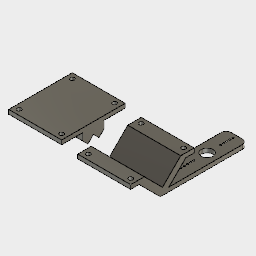
pen-arm (Autodesk Fusion 360 design; units mm, degrees)
Autodesk Fusion 360 part; units mm, degrees
sketch "Sketch1" plane through (0, 0, 0) normal (0, 0, 1) x (1, 0, 0)
  line L0 (-10, -50) -> (10, -50)
  line L1 (10, -50) -> (10, 45)
  line L2 (5, 50) -> (-5, 50)
  line L3 (-10, 45) -> (-10, -50)
  line L4 (-10, -50) -> (10, 50) construction
  line L5 (10, -50) -> (-10, 50) construction
  circle A0 centre (0.0086, 22) radius 5.5
  circle A1 centre (0.0086, 34.5) radius 0.75
  circle A2 centre (0.0086, 37.5) radius 0.75
  circle A3 centre (0.0086, 40.5) radius 0.75
  circle A4 centre (0.0086, 43.5) radius 0.75
  circle A5 centre (0.0086, 46.5) radius 0.75
  arc A6 (10, 45) -> (5, 50) centre (5, 45) ccw
  arc A7 (-5, 50) -> (-10, 45) centre (-5, 45) ccw
  circle A8 centre (0.0086, 9.5) radius 0.75
  circle A9 centre (0.0086, 6.5) radius 0.75
  circle A10 centre (0.0086, 3.5) radius 0.75
  circle A11 centre (0.0086, 0.5) radius 0.75
  circle A12 centre (0.0086, -2.5) radius 0.75
  dimension "d1" = 20
  dimension "d2" = 100
  dimension "d3" = 11
  dimension "d4" = 28
  dimension "d5" = 1.5
  dimension "d6" = 12.5
  dimension "d7" = 1.5
  dimension "d8" = 3
  dimension "d9" = 1.5
  dimension "d10" = 3
  dimension "d11" = 1.5
  dimension "d12" = 3
  dimension "d13" = 1.5
  dimension "d14" = 3
  dimension "d15" = 5
  dimension "d16" = 5
  dimension "d17" = 1.5
  dimension "d18" = 12.5
  dimension "d19" = 1.5
  dimension "d20" = 1.5
  dimension "d21" = 1.5
  dimension "d22" = 1.5
  dimension "d23" = 3
  dimension "d24" = 3
  dimension "d25" = 3
  dimension "d26" = 3
  measures "d1" distance of L4.end L5.end
  measures "d2" distance of L0.end L4.end
  measures "d3" diameter of A0
  measures "d4" distance of L2 A0.centre
  measures "d5" diameter of A1
  measures "d6" distance of A0.centre A1.centre
  measures "d7" diameter of A2
  measures "d8" distance of A1.centre A2.centre
  measures "d9" diameter of A3
  measures "d10" distance of A2.centre A3.centre
  measures "d11" diameter of A4
  measures "d12" distance of A3.centre A4.centre
  measures "d13" diameter of A5
  measures "d14" distance of A4.centre A5.centre
  measures "d15" radius of A6
  measures "d16" radius of A7
  measures "d17" diameter of A8
  measures "d18" distance of A0.centre A8.centre
  measures "d19" diameter of A9
  measures "d20" diameter of A10
  measures "d21" diameter of A11
  measures "d22" diameter of A12
  measures "d23" distance of A8.centre A9.centre
  measures "d24" distance of A9.centre A10.centre
  measures "d25" distance of A10.centre A11.centre
  measures "d26" distance of A11.centre A12.centre
extrude "Extrude1" add sketch "Sketch1" along normal blind 4 makes body 1
sketch "Sketch2" plane through (-10, 0, 0) normal (-1, 0, 0) x (0, -1, 0)
  line L0 (-45, 0) -> (50, 0)
  line L1 (50, 0) -> (50, 4)
  line L2 (50, 4) -> (-45, 4)
  line L3 (-45, 4) -> (-45, 0)
  line L4 (50, 4) -> (10, 4)
  line L5 (10, 4) -> (10, 0)
  line L6 (10, 0) -> (50, 0)
  line L7 (50, 0) -> (50, 4)
  dimension "d31" = 40
  measures "d31" distance of L1.end L4.end
extrude "Extrude2" add sketch "Sketch2" along normal blind 30 contours L0 L1 L2 L4 L5 L6 L7 bodies 1
sketch "Sketch3" plane through (0, 0, 4) normal (0, 0, 1) x (-1, 0, 0)
  circle A0 centre (-0.0086, -0.5) radius 0.75
  circle A1 centre (-0.0086, -34.5) radius 0.75
  circle A2 centre (-0.0086, -37.5) radius 0.75
  circle A3 centre (-0.0086, -40.5) radius 0.75
  circle A4 centre (-0.0086, -6.5) radius 0.75
  circle A5 centre (-0.0086, -46.5) radius 0.75
  circle A6 centre (-0.0086, -43.5) radius 0.75
  circle A7 centre (-0.0086, -9.5) radius 0.75
  circle A8 centre (-0.0086, -22) radius 5.5
  circle A9 centre (-0.0086, 2.5) radius 0.75
  circle A10 centre (-0.0086, -3.5) radius 0.75
  arc A11 (5, -50) -> (10, -45) centre (5, -45) ccw
  line L0 (10, -45) -> (10, 10)
  line L1 (10, 10) -> (40, 10)
  line L2 (40, 10) -> (40, 50)
  line L3 (40, 50) -> (-10, 50)
  line L4 (-10, 50) -> (-10, -45)
  arc A12 (-10, -45) -> (-5, -50) centre (-5, -45) ccw
  line L5 (-5, -50) -> (5, -50)
  line L6 (-10, 50) -> (40, 50)
  line L7 (40, 50) -> (40, 10)
  line L8 (40, 10) -> (-10, 10)
  line L9 (-10, 10) -> (-10, 50)
extrude "Extrude3" add sketch "Sketch3" along normal blind 20 contours L1 L2 L3 L4 L6 L7 L8 L9 bodies 1
sketch "Sketch4" plane through (0, 0, 24) normal (0, 0, 1) x (-1, 0, 0)
  line L0 (-10, 10) -> (40, 10)
  line L1 (40, 10) -> (40, 50)
  line L2 (40, 50) -> (-10, 50)
  line L3 (-10, 50) -> (-10, 10)
  line L4 (40, 30) -> (-10, 30)
split "Split1" by curves path "Sketch4" along L4 bodies 1 makes body 2 at (-6.6667, -50, 16)
draft "Draft1" angle -45 neutral plane through (-40, -50, 4) pull (0, -1, 0) 1 faces at (-6.6667, -43.3333, 24) on bodies 2
draft "Draft2" angle -45 neutral plane through (-10, -10, 4) pull (0, 1, 0) 1 faces at (-6.6667, -23.3333, 24) on bodies 1
combine "Combine1" operation add target body 2 tool bodies 1
sketch "Sketch5" plane through (0, -10, 0) normal (0, 1, 0) x (-1, 0, 0)
  line L0 (10, 4) -> (10, 0)
  line L1 (10, 0) -> (40, 0)
  line L2 (40, 0) -> (40, 24)
  line L3 (40, 24) -> (-10, 24)
  line L4 (-10, 24) -> (-10, 4)
  line L5 (-10, 4) -> (10, 4)
  line L6 (-10, 24) -> (40, 24)
  line L7 (40, 24) -> (40, 20)
  line L8 (40, 20) -> (-10, 20)
  line L9 (-10, 20) -> (-10, 24)
  dimension "d40" = 4
  measures "d40" distance of L3.end L8.end
extrude "Extrude4" add sketch "Sketch5" along normal blind 10 contours L2 L3 L4 L6 L7 L8 L9 bodies 2
sketch "Sketch6" plane through (0, -50, 0) normal (0, -1, 0) x (1, 0, 0)
  line L0 (-40, 0) -> (10, 0)
  line L1 (10, 0) -> (10, 24)
  line L2 (10, 24) -> (-40, 24)
  line L3 (-40, 24) -> (-40, 0)
  line L4 (-40, 24) -> (10, 24)
  line L5 (10, 24) -> (10, 20)
  line L6 (10, 20) -> (-40, 20)
  line L7 (-40, 20) -> (-40, 24)
  dimension "d43" = 4
  measures "d43" distance of L2.end L6.end
extrude "Extrude5" add sketch "Sketch6" along normal blind 10 contours L1 L2 L3 L4 L5 L6 L7 bodies 2
chamfer "Chamfer1" distance 2 angle 45 1 edges at (-15, -10, 20) on bodies 2
chamfer "Chamfer2" distance 2 angle 45 1 edges at (-15, -50, 20) on bodies 2
sketch "Sketch7" plane through (0, 0, 0) normal (0, 0, 1) x (1, 0, 0)
  line L0 (-49.9475, -0.0799) -> (-99.9475, -0.0799)
  line L1 (-99.9475, -0.0799) -> (-99.9475, -60.0799)
  line L2 (-99.9475, -60.0799) -> (-49.9475, -60.0799)
  line L3 (-49.9475, -60.0799) -> (-49.9475, -0.0799)
  dimension "d48" = 50
  dimension "d49" = 60
  measures "d48" distance of L0.start L0.end
  measures "d49" distance of L0.start L2.end
extrude "Extrude6" add sketch "Sketch7" along normal blind 4 separate body makes body 3
sketch "Sketch8" plane through (0, 0, 4) normal (0, 0, 1) x (-1, 0, 0)
  line L0 (49.9475, 60.0799) -> (49.9475, 0.0799)
  line L1 (49.9475, 0.0799) -> (99.9475, 0.0799)
  line L2 (99.9475, 0.0799) -> (99.9475, 60.0799)
  line L3 (99.9475, 60.0799) -> (49.9475, 60.0799)
  line L4 (99.9475, 30.0799) -> (49.9475, 30.0799)
  line L5 (99.9475, 40.0799) -> (49.9475, 40.0799)
  line L6 (99.9475, 20.0799) -> (49.9475, 20.0799)
  dimension "d52" = 10
  dimension "d53" = 10
  measures "d52" distance of L4 L5
  measures "d53" distance of L4 L6
extrude "Extrude7" add sketch "Sketch8" along normal blind 10 contours L0 L2 L4 L5 bodies 3
chamfer "Chamfer3" distance 7 angle 45 1 edges at (-74.9475, -30.0799, 14) on bodies 3
extrude "Extrude8" add sketch "Sketch8" along normal blind 10 contours L0 L2 L4 L6 bodies 3
chamfer "Chamfer4" distance 7 angle 45 1 edges at (-74.9475, -30.0799, 14) on bodies 3
sketch "Sketch9" plane through (0, 0, 24) normal (0, 0, 1) x (-1, 0, 0)
  line L0 (40, 10) -> (-10, 10)
  line L1 (-10, 10) -> (-10, 0)
  line L2 (-10, 0) -> (40, 0)
  line L3 (40, 0) -> (40, 10)
  circle A0 centre (-5, 5) radius 2
  circle A1 centre (35, 5) radius 2
  circle A2 centre (35, 55) radius 2
  circle A3 centre (-5, 55) radius 2
  circle A4 centre (54.9475, 5.0799) radius 2
  circle A5 centre (94.9475, 5.0799) radius 2
  circle A6 centre (94.9475, 55.0799) radius 2
  circle A7 centre (54.9475, 55.0799) radius 2
  line L4 (-10, 60) -> (40, 60)
  line L5 (40, 50) -> (40, 60)
  line L6 (-10, 50) -> (-10, 60)
  line L7 (99.9475, 60.0799) -> (49.9475, 60.0799)
  line L8 (99.9475, 0.0799) -> (99.9475, 60.0799)
  line L9 (49.9475, 60.0799) -> (49.9475, 0.0799)
  line L10 (49.9475, 0.0799) -> (99.9475, 0.0799)
  dimension "d60" = 4
  dimension "d61" = 4
  dimension "d62" = 4
  dimension "d63" = 4
  dimension "d64" = 4
  dimension "d65" = 4
  dimension "d66" = 4
  dimension "d67" = 4
  dimension "d68" = 5
  dimension "d69" = 5
  dimension "d70" = 5
  dimension "d71" = 5
  dimension "d72" = 5
  dimension "d73" = 5
  dimension "d74" = 5
  dimension "d75" = 5
  dimension "d76" = 5
  dimension "d77" = 5
  dimension "d78" = 5
  dimension "d79" = 5
  dimension "d80" = 5
  dimension "d81" = 5
  dimension "d82" = 5
  dimension "d83" = 5
  measures "d60" diameter of A0
  measures "d61" diameter of A1
  measures "d62" diameter of A2
  measures "d63" diameter of A3
  measures "d64" diameter of A4
  measures "d65" diameter of A5
  measures "d66" diameter of A6
  measures "d67" diameter of A7
  measures "d68" distance of L2 A1.centre
  measures "d69" distance of L3 A1.centre
  measures "d70" distance of L2 A0.centre
  measures "d71" distance of L1 A0.centre
  measures "d72" distance of A2.centre L4
  measures "d73" distance of A2.centre L5
  measures "d74" distance of A3.centre L4
  measures "d75" distance of A3.centre L6
  measures "d76" distance of A6.centre L7
  measures "d77" distance of A6.centre L8
  measures "d78" distance of A7.centre L9
  measures "d79" distance of A7.centre L7
  measures "d80" distance of A4.centre L9
  measures "d81" distance of A4.centre L10
  measures "d82" distance of A5.centre L10
  measures "d83" distance of A5.centre L8
extrude "Extrude9" cut sketch "Sketch9" against normal blind 31 contours A2 bodies 2
extrude "Extrude10" cut sketch "Sketch9" against normal blind 20 contours A3 bodies 2
extrude "Extrude11" cut sketch "Sketch9" against normal blind 20 contours A0 bodies 2
extrude "Extrude12" cut sketch "Sketch9" against normal blind 10 contours A1 bodies 2
extrude "Extrude13" cut sketch "Sketch9" against normal blind 33 contours A5 bodies 3
extrude "Extrude14" cut sketch "Sketch9" against normal blind 42 contours A4 bodies 3
extrude "Extrude15" cut sketch "Sketch9" against normal blind 43 contours A7 bodies 3
extrude "Extrude16" cut sketch "Sketch9" against normal blind 35 contours A6 bodies 3
move_body "Move1" bodies 3 to x (1, 0, 0) y (0, -1, 0) z (0, 0, -1) at (-5, -60.1598, 28)
chamfer "Chamfer5" distance 3 angle 45 1 edges at (-79.9475, -20.0799, 14) on bodies 3
chamfer "Chamfer6" distance 3 angle 45 1 edges at (-79.9475, -40.0799, 14) on bodies 3
move_face "OffsetFaces1" offset 2 1 faces at (-6.6667, -16.6667, 17.3333) on bodies 2
move_face "OffsetFaces2" offset 2 1 faces at (-23.3333, -37.6095, 11.6095) on bodies 2
chamfer "Chamfer7" distance 18 angle 45 1 edges at (-15, -50, 0) on bodies 2
chamfer "Chamfer8" distance 18 angle 45 1 edges at (-25, -10, 0) on bodies 2
move_face "OffsetFaces3" offset 2.5 3 faces at (-71.6142, -37.079, 14) (-88.2809, -32.4128, 18.6657) (-88.2809, -30.0799, 20.9995) on bodies 3
move_face "OffsetFaces4" offset 2.5 2 faces at (-71.6142, -26.5676, 17.4877) (-71.6142, -23.0795, 14) on bodies 3
